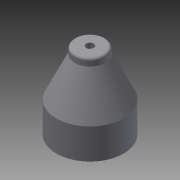
# Autodesk Inventor part: brush fitting parta
Saved by Autodesk Inventor 2013 SP2 (Build 170200200, 200)
## iProperties
Created: 2017-05-15
Part Number: brush fitting parta
Material: Generic
Document SubType Name: Modeling
Designer: Herman de Vries
Density: 1 g/cm^3
Author: Herman de Vries
Autodesk Inventor part; units mm, degrees
ref_plane "YZ Plane" through (0, 0, 0) normal (1, 0, 0) x (0, 1, 0)
ref_plane "XZ Plane" through (0, 0, 0) normal (0, 1, 0) x (-1, 0, 0)
ref_plane "XY Plane" through (0, 0, 0) normal (0, 0, 1) x (1, 0, 0)
sketch "Sketch1" plane through (0, 0, 0) normal (1, 0, 0) x (0, 1, 0)
  line L0 (0, 16) -> (2.5, 16) construction
  arc A0 (9.9609, 0) -> (2.5, 16) centre (-28.1983, -8.0544) ccw construction
  line L1 (0, 12) -> (0, 0) construction
  line L2 (2.5, 16) -> (2.5, 16) construction
  line L3 (9.9609, 0) -> (4.5, 0) construction
  line L4 (4.5, 9) -> (0, 9)
  line L5 (4.5, 9) -> (4.5, 0)
  line L6 (0, 12) -> (0, 9)
  line L7 (9.9609, 0) -> (2.5, 16) construction
  line L8 (3.2, 14.4988) -> (3.2, 16)
  line L9 (3.2, 16) -> (2.5, 16)
  line L10 (7, 0) -> (7, 6.3497)
  line L11 (4.5, 0) -> (7, 0)
  line L12 (7, 6.3497) -> (3.2, 14.4988)
  line L13 (0, 12) -> (0.8, 12)
  line L14 (0.8, 12) -> (0.8, 16)
  line L15 (2.5, 16) -> (0.8, 16)
  dimension "d0" = 2.5
  dimension "d5" = 4.5
  dimension "d11" = 9
  dimension "d12" = 16
  dimension "d13" = 115
  dimension "d14" = 3.2
  dimension "d18" = 1.5011
  dimension "d19" = 8.1491
  dimension "d20" = 7
  dimension "d21" = 4
  dimension "d22" = 0.8
  constraints: 32 end point, 5 point on line, 4 collinear, 3 parallel, 3 perpendicular, 2 point on circle, 1 centre point, 1 horizontal, 1 horizontal alignment, 1 vertical, 1 vertical alignment
  measures "d0" distance of L0.start L0.end
  measures "d5" distance of L4.start L4.end
  measures "d11" distance from line of L4 L1.end
  measures "d12" distance from line of L0 L1.end
  measures "d13" angle of L3 L7
  measures "d14" distance from line of L0.start L8
  measures "d18" distance of L8.start L8.end
  measures "d19" vertical distance of L10.end L8.start
  measures "d20" distance of L10.start L1.end
  measures "d21" distance of L13.end L14.end
  measures "d22" distance of L1.start L13.end
revolve "Revolution1" add sketch "Sketch1" angle 360 about axis through (0, 0, 12) along (0, 0, -1)
sketch "Sketch2" plane through (0, 0, 0) normal (1, 0, 0) x (0, 1, 0)
  arc A0 (-2.5, 15) -> (2.5, 15) centre (0, 15) ccw projected
  circle A1 centre (0, 15) radius 1.5
  line L0 (0.6744, 16.3398) -> (-0.6744, 13.6602)
  point P0 (0, 0)
  dimension "d8" = 3
  constraints: 2 end point, 2 point on circle, 1 centre point, 1 coincident, 1 midpoint
  measures "d8" diameter of A1
revolve "Revolution2" [suppressed]
fillet "Fillet1" radius 0.5 2 edges at (0, -3.2, 16) (0, -4.5, 9)
body "Solid1"
